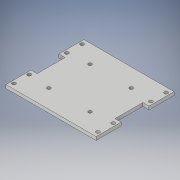
# Autodesk Inventor part: 000.104 - Дно цетрального сегмента
Saved by Autodesk Inventor 2019 (Build 230136000, 136)
## iProperties
Created: 2020-06-06
Part Number: 000.104 - Дно цетрального сегмента
Material: Типовые
Document SubType Name: Modeling
Designer: Петров Иван
Density: 1 g/cm^3
Appearance: По умолчанию
Author: Петров Иван
Autodesk Inventor part; units mm, degrees
ref_plane "YZ Plane" through (0, 0, 0) normal (1, 0, 0) x (0, 1, 0)
ref_plane "XZ Plane" through (0, 0, 0) normal (0, 1, 0) x (-1, 0, 0)
ref_plane "XY Plane" through (0, 0, 0) normal (0, 0, 1) x (1, 0, 0)
sketch "Эскиз1" plane through (0, 0, 0) normal (0, 1, 0) x (-1, 0, 0)
  circle A0 centre (-37.75, 16.875) radius 1.6
  circle A1 centre (-37.75, 30.625) radius 1.6
  line L0 (-40.5, 35) -> (-40.5, 12.5)
  line L1 (-40.5, 12.5) -> (-35, 12.5)
  line L2 (-35, 35) -> (-35, 12.5)
  line L3 (-35, 35) -> (-40.5, 35)
  circle A2 centre (37.75, 16.875) radius 1.6
  circle A3 centre (37.75, 30.625) radius 1.6
  line L4 (40.5, 35) -> (40.5, 12.5)
  line L5 (35, 35) -> (40.5, 35)
  line L6 (35, 12.5) -> (35, 35)
  line L7 (40.5, 12.5) -> (35, 12.5)
  circle A4 centre (37.75, -16.875) radius 1.6
  circle A5 centre (37.75, -30.625) radius 1.6
  line L8 (40.5, -35) -> (35, -35)
  line L9 (40.5, -12.5) -> (40.5, -35)
  line L10 (35, -12.5) -> (40.5, -12.5)
  line L11 (35, -35) -> (35, -12.5)
  circle A6 centre (-37.75, -16.875) radius 1.6
  circle A7 centre (-37.75, -30.625) radius 1.6
  line L12 (-40.5, -35) -> (-35, -35)
  line L13 (-35, -12.5) -> (-35, -35)
  line L14 (-35, -12.5) -> (-40.5, -12.5)
  line L15 (-40.5, -12.5) -> (-40.5, -35)
  line L16 (-40.5, -12.5) -> (-35, -12.5)
  line L17 (-35, 12.5) -> (-35, -12.5)
  line L18 (-35, 12.5) -> (-40.5, 12.5)
  line L19 (-40.5, -12.5) -> (-40.5, 12.5)
  line L20 (40.5, 12.5) -> (35, 12.5)
  line L21 (35, -12.5) -> (35, 12.5)
  line L22 (35, -12.5) -> (40.5, -12.5)
  line L23 (40.5, -12.5) -> (40.5, 12.5)
  line L24 (20, 35) -> (-20, 35)
  line L25 (-20, 35) -> (-35, 35)
  line L26 (35, 35) -> (20, 35)
  line L27 (-35, -35) -> (-20, -35)
  line L28 (-20, -35) -> (20, -35)
  line L29 (20, -35) -> (35, -35)
  line L30 (40.5, 35) -> (-40.5, 35)
  line L31 (-40.5, 35) -> (-40.5, -35)
  line L32 (-40.5, -35) -> (40.5, -35)
  line L33 (40.5, -35) -> (40.5, 35)
  point P0 (0, 0)
  point P1 (0, 0)
  constraints: 68 end point, 8 centre point, 2 parallel, 1 horizontal, 1 perpendicular
extrude "Выдавливание1" add sketch "Эскиз1" along normal blind 3 contours L3 L2 L1 L0 | L25 L24 L26 L6 L21 L11 L29 L28 L27 L13 L17 L2 | L14 L13 L12 L15 | L5 L4 L7 L6 | L10 L9 L8 L11
sketch "Эскиз2" plane through (0, 3, 0) normal (0, 1, 0) x (1, 0, 0)
  line L0 (21.5, 21.875) -> (21.5, -21.875)
  line L1 (-21.5, 21.875) -> (21.5, 21.875)
  line L2 (-21.5, -21.875) -> (-21.5, 21.875)
  line L3 (21.5, -21.875) -> (-21.5, -21.875)
  circle A0 centre (-18.5, 18.5) radius 1.5
  circle A1 centre (18.5, 18.5) radius 1.5
  circle A2 centre (18.5, -18.5) radius 1.5
  circle A3 centre (-18.5, -18.5) radius 1.5
  point P0 (0, 0)
  point P1 (0, 0)
  constraints: 8 end point, 4 centre point
extrude "Выдавливание2" cut sketch "Эскиз2" against normal blind 10 contours A0 | A1 | A2 | A3
